Autodesk Inventor part; units mm, degrees
(part 2 of 2)
sketch "Sketch100" plane through (-49.2721, -156.6302, 132.2833) normal (0, -0.6427876, 0.7660444) x (1, 0, 0)
  line L0 (3.9589, -29.4362) -> (45.851, -29.4362) construction
  line L1 (45.851, -29.4362) -> (45.851, -41.0729) construction
  line L2 (45.851, -41.0729) -> (3.9589, -41.0729) construction
  line L3 (3.9589, -41.0729) -> (3.9589, -29.4362) construction
  spline S0 degree 2 poles (6.671, -31.0269) (6.671, -31.4443) (6.3326, -32.1162) (6.0486, -32.3039) knots 0 0 0 1 2 2 2
  spline S1 degree 2 poles (6.0486, -32.3039) (5.8164, -32.4496) (5.3397, -32.5484) (4.9692, -32.5484) knots 0 0 0 1 2 2 2
  line L4 (4.9692, -32.5484) -> (4.2677, -32.5484)
  line L5 (4.2677, -32.5484) -> (4.2677, -29.5004)
  line L6 (4.2677, -29.5004) -> (4.9617, -29.5004)
  spline S2 degree 2 poles (4.9617, -29.5004) (5.3915, -29.5004) (5.8806, -29.6289) (6.0535, -29.7425) knots 0 0 0 1 2 2 2
  spline S3 degree 2 poles (6.0535, -29.7425) (6.3474, -29.9376) (6.671, -30.5823) (6.671, -31.0269) knots 0 0 0 1 2 2 2
  spline S4 degree 2 poles (6.2486, -31.0219) (6.2486, -30.6712) (6.0164, -30.1747) (5.7867, -30.0339) knots 0 0 0 1 2 2 2
  spline S5 degree 2 poles (5.7867, -30.0339) (5.6237, -29.9376) (5.2557, -29.8512) (4.9815, -29.8512) knots 0 0 0 1 2 2 2
  line L7 (4.9815, -29.8512) -> (4.6728, -29.8512)
  line L8 (4.6728, -29.8512) -> (4.6728, -32.1977)
  line L9 (4.6728, -32.1977) -> (4.9815, -32.1977)
  spline S6 degree 2 poles (4.9815, -32.1977) (5.2507, -32.1977) (5.6583, -32.1112) (5.8238, -31.9951) knots 0 0 0 1 2 2 2
  spline S7 degree 2 poles (5.8238, -31.9951) (6.0362, -31.8519) (6.2486, -31.3776) (6.2486, -31.0219) knots 0 0 0 1 2 2 2
  spline S8 degree 2 poles (8.1752, -32.6126) (7.906, -32.6126) (7.5059, -32.4718) (7.3651, -32.331) knots 0 0 0 1 2 2 2
  spline S9 degree 2 poles (7.3651, -32.331) (7.2045, -32.173) (7.0736, -31.7284) (7.0736, -31.4023) knots 0 0 0 1 2 2 2
  line L10 (7.0736, -31.4023) -> (7.0736, -29.5004)
  line L11 (7.0736, -29.5004) -> (7.4787, -29.5004)
  line L12 (7.4787, -29.5004) -> (7.4787, -31.4023)
  spline S10 degree 2 poles (7.4787, -31.4023) (7.4787, -31.6147) (7.533, -31.9013) (7.6096, -32.0174) knots 0 0 0 1 2 2 2
  spline S11 degree 2 poles (7.6096, -32.0174) (7.6911, -32.1409) (7.9727, -32.2668) (8.1752, -32.2668) knots 0 0 0 1 2 2 2
  spline S12 degree 2 poles (8.1752, -32.2668) (8.3654, -32.2668) (8.6618, -32.1409) (8.7433, -32.0174) knots 0 0 0 1 2 2 2
  spline S13 degree 2 poles (8.7433, -32.0174) (8.8199, -31.9013) (8.8743, -31.6172) (8.8743, -31.4122) knots 0 0 0 1 2 2 2
  line L13 (8.8743, -31.4122) -> (8.8743, -29.5004)
  line L14 (8.8743, -29.5004) -> (9.2793, -29.5004)
  line L15 (9.2793, -29.5004) -> (9.2793, -31.4023)
  spline S14 degree 2 poles (9.2793, -31.4023) (9.2793, -31.721) (9.1509, -32.1754) (8.9879, -32.331) knots 0 0 0 1 2 2 2
  spline S15 degree 2 poles (8.9879, -32.331) (8.8421, -32.4743) (8.4568, -32.6126) (8.1752, -32.6126) knots 0 0 0 1 2 2 2
  line L16 (9.5313, -32.5484) -> (10.5588, -29.5004)
  line L17 (10.5588, -29.5004) -> (11.0577, -29.5004)
  line L18 (11.0577, -29.5004) -> (12.0853, -32.5484)
  line L19 (12.0853, -32.5484) -> (11.658, -32.5484)
  line L20 (11.658, -32.5484) -> (11.3813, -31.6963)
  line L21 (11.3813, -31.6963) -> (10.2179, -31.6963)
  line L22 (10.2179, -31.6963) -> (9.9413, -32.5484)
  line L23 (9.9413, -32.5484) -> (9.5313, -32.5484)
  line L24 (11.2702, -31.3505) -> (10.7984, -29.9154)
  line L25 (10.7984, -29.9154) -> (10.3291, -31.3505)
  line L26 (10.3291, -31.3505) -> (11.2702, -31.3505)
  line L27 (14.1403, -32.5484) -> (12.3743, -32.5484)
  line L28 (12.3743, -32.5484) -> (12.3743, -29.5004)
  line L29 (12.3743, -29.5004) -> (12.7793, -29.5004)
  line L30 (12.7793, -29.5004) -> (12.7793, -32.1878)
  line L31 (12.7793, -32.1878) -> (14.1403, -32.1878)
  line L32 (14.1403, -32.1878) -> (14.1403, -32.5484)
  line L33 (17.9787, -29.5004) -> (16.929, -32.5484)
  line L34 (16.929, -32.5484) -> (16.4918, -32.5484)
  line L35 (16.4918, -32.5484) -> (15.442, -29.5004)
  line L36 (15.442, -29.5004) -> (15.8767, -29.5004)
  line L37 (15.8767, -29.5004) -> (16.7215, -32.0322)
  line L38 (16.7215, -32.0322) -> (17.5662, -29.5004)
  line L39 (17.5662, -29.5004) -> (17.9787, -29.5004)
  line L40 (19.3323, -32.5484) -> (18.1516, -32.5484)
  line L41 (18.1516, -32.5484) -> (18.1516, -32.2372)
  line L42 (18.1516, -32.2372) -> (18.5394, -32.2372)
  line L43 (18.5394, -32.2372) -> (18.5394, -29.8116)
  line L44 (18.5394, -29.8116) -> (18.1516, -29.8116)
  line L45 (18.1516, -29.8116) -> (18.1516, -29.5004)
  line L46 (18.1516, -29.5004) -> (19.3323, -29.5004)
  line L47 (19.3323, -29.5004) -> (19.3323, -29.8116)
  line L48 (19.3323, -29.8116) -> (18.9445, -29.8116)
  line L49 (18.9445, -29.8116) -> (18.9445, -32.2372)
  line L50 (18.9445, -32.2372) -> (19.3323, -32.2372)
  line L51 (19.3323, -32.2372) -> (19.3323, -32.5484)
  spline S16 degree 2 poles (20.6834, -32.6028) (20.3524, -32.6028) (19.8881, -32.4644) (19.683, -32.3656) knots 0 0 0 1 2 2 2
  line L52 (19.683, -32.3656) -> (19.683, -31.8568)
  line L53 (19.683, -31.8568) -> (19.7127, -31.8568)
  spline S17 degree 2 poles (19.7127, -31.8568) (19.9128, -32.0445) (20.4191, -32.252) (20.6538, -32.252) knots 0 0 0 1 2 2 2
  spline S18 degree 2 poles (20.6538, -32.252) (20.9897, -32.252) (21.333, -31.9729) (21.333, -31.7432) knots 0 0 0 1 2 2 2
  spline S19 degree 2 poles (21.333, -31.7432) (21.333, -31.5604) (21.1527, -31.3332) (20.9576, -31.2764) knots 0 0 0 1 2 2 2
  spline S20 degree 2 poles (20.9576, -31.2764) (20.8168, -31.2368) (20.5821, -31.1825) (20.4068, -31.138) knots 0 0 0 1 2 2 2
  spline S21 degree 2 poles (20.4068, -31.138) (20.2487, -31.096) (19.9992, -30.9701) (19.9029, -30.8688) knots 0 0 0 1 2 2 2
  spline S22 degree 2 poles (19.9029, -30.8688) (19.809, -30.7675) (19.7053, -30.4958) (19.7053, -30.318) knots 0 0 0 1 2 2 2
  spline S23 degree 2 poles (19.7053, -30.318) (19.7053, -29.9475) (20.2833, -29.4461) (20.7303, -29.4461) knots 0 0 0 1 2 2 2
  spline S24 degree 2 poles (20.7303, -29.4461) (20.9872, -29.4461) (21.4417, -29.5473) (21.6368, -29.6437) knots 0 0 0 1 2 2 2
  line L54 (21.6368, -29.6437) -> (21.6368, -30.1278)
  line L55 (21.6368, -30.1278) -> (21.6072, -30.1278)
  spline S25 degree 2 poles (21.6072, -30.1278) (21.4615, -29.9944) (21.007, -29.7968) (20.7575, -29.7968) knots 0 0 0 1 2 2 2
  spline S26 degree 2 poles (20.7575, -29.7968) (20.4759, -29.7968) (20.1276, -30.0611) (20.1276, -30.276) knots 0 0 0 1 2 2 2
  spline S27 degree 2 poles (20.1276, -30.276) (20.1276, -30.4687) (20.3327, -30.6984) (20.5253, -30.7502) knots 0 0 0 1 2 2 2
  spline S28 degree 2 poles (20.5253, -30.7502) (20.6538, -30.7848) (21.0267, -30.8737) (21.1502, -30.9108) knots 0 0 0 1 2 2 2
  spline S29 degree 2 poles (21.1502, -30.9108) (21.4639, -31.0071) (21.7554, -31.3949) (21.7554, -31.679) knots 0 0 0 1 2 2 2
  spline S30 degree 2 poles (21.7554, -31.679) (21.7554, -31.8593) (21.6097, -32.2051) (21.4787, -32.3261) knots 0 0 0 1 2 2 2
  spline S31 degree 2 poles (21.4787, -32.3261) (21.333, -32.4595) (20.9625, -32.6028) (20.6834, -32.6028) knots 0 0 0 1 2 2 2
  line L56 (23.23, -32.5484) -> (22.0493, -32.5484)
  line L57 (22.0493, -32.5484) -> (22.0493, -32.2372)
  line L58 (22.0493, -32.2372) -> (22.4371, -32.2372)
  line L59 (22.4371, -32.2372) -> (22.4371, -29.8116)
  line L60 (22.4371, -29.8116) -> (22.0493, -29.8116)
  line L61 (22.0493, -29.8116) -> (22.0493, -29.5004)
  line L62 (22.0493, -29.5004) -> (23.23, -29.5004)
  line L63 (23.23, -29.5004) -> (23.23, -29.8116)
  line L64 (23.23, -29.8116) -> (22.8422, -29.8116)
  line L65 (22.8422, -29.8116) -> (22.8422, -32.2372)
  line L66 (22.8422, -32.2372) -> (23.23, -32.2372)
  line L67 (23.23, -32.2372) -> (23.23, -32.5484)
  spline S32 degree 2 poles (25.8877, -29.8487) (26.0606, -30.0512) (26.2533, -30.644) (26.2533, -31.0244) knots 0 0 0 1 2 2 2
  spline S33 degree 2 poles (26.2533, -31.0244) (26.2533, -31.3949) (26.0656, -31.9951) (25.8877, -32.1977) knots 0 0 0 1 2 2 2
  spline S34 degree 2 poles (25.8877, -32.1977) (25.7, -32.4101) (25.2035, -32.6126) (24.9047, -32.6126) knots 0 0 0 1 2 2 2
  spline S35 degree 2 poles (24.9047, -32.6126) (24.5959, -32.6126) (24.1019, -32.4027) (23.9216, -32.1977) knots 0 0 0 1 2 2 2
  spline S36 degree 2 poles (23.9216, -32.1977) (23.7462, -31.9951) (23.5585, -31.3999) (23.5585, -31.0244) knots 0 0 0 1 2 2 2
  spline S37 degree 2 poles (23.5585, -31.0244) (23.5585, -30.6416) (23.7487, -30.0586) (23.9241, -29.8487) knots 0 0 0 1 2 2 2
  spline S38 degree 2 poles (23.9241, -29.8487) (24.1019, -29.6461) (24.5984, -29.4362) (24.9047, -29.4362) knots 0 0 0 1 2 2 2
  spline S39 degree 2 poles (24.9047, -29.4362) (25.2159, -29.4362) (25.7148, -29.6536) (25.8877, -29.8487) knots 0 0 0 1 2 2 2
  spline S40 degree 2 poles (25.8309, -31.0244) (25.8309, -30.7231) (25.7, -30.2562) (25.5814, -30.1031) knots 0 0 0 1 2 2 2
  spline S41 degree 2 poles (25.5814, -30.1031) (25.4604, -29.945) (25.1195, -29.7869) (24.9071, -29.7869) knots 0 0 0 1 2 2 2
  spline S42 degree 2 poles (24.9071, -29.7869) (24.6873, -29.7869) (24.3563, -29.9401) (24.2303, -30.1031) knots 0 0 0 1 2 2 2
  spline S43 degree 2 poles (24.2303, -30.1031) (24.1093, -30.2587) (23.9809, -30.728) (23.9809, -31.0244) knots 0 0 0 1 2 2 2
  spline S44 degree 2 poles (23.9809, -31.0244) (23.9809, -31.6246) (24.4848, -32.2619) (24.9071, -32.2619) knots 0 0 0 1 2 2 2
  spline S45 degree 2 poles (24.9071, -32.2619) (25.3295, -32.2619) (25.8309, -31.6246) (25.8309, -31.0244) knots 0 0 0 1 2 2 2
  line L68 (28.8789, -32.5484) -> (28.4244, -32.5484)
  line L69 (28.4244, -32.5484) -> (27.0758, -29.9203)
  line L70 (27.0758, -29.9203) -> (27.0758, -32.5484)
  line L71 (27.0758, -32.5484) -> (26.6979, -32.5484)
  line L72 (26.6979, -32.5484) -> (26.6979, -29.5004)
  line L73 (26.6979, -29.5004) -> (27.2734, -29.5004)
  line L74 (27.2734, -29.5004) -> (28.501, -31.9136)
  line L75 (28.501, -31.9136) -> (28.501, -29.5004)
  line L76 (28.501, -29.5004) -> (28.8789, -29.5004)
  line L77 (28.8789, -29.5004) -> (28.8789, -32.5484)
  line L78 (33.0187, -32.5484) -> (32.6136, -32.5484)
  line L79 (32.6136, -32.5484) -> (32.6136, -31.0565)
  line L80 (32.6136, -31.0565) -> (31.2106, -31.0565)
  line L81 (31.2106, -31.0565) -> (31.2106, -32.5484)
  line L82 (31.2106, -32.5484) -> (30.8055, -32.5484)
  line L83 (30.8055, -32.5484) -> (30.8055, -29.5004)
  line L84 (30.8055, -29.5004) -> (31.2106, -29.5004)
  line L85 (31.2106, -29.5004) -> (31.2106, -30.6959)
  line L86 (31.2106, -30.6959) -> (32.6136, -30.6959)
  line L87 (32.6136, -30.6959) -> (32.6136, -29.5004)
  line L88 (32.6136, -29.5004) -> (33.0187, -29.5004)
  line L89 (33.0187, -29.5004) -> (33.0187, -32.5484)
  spline S46 degree 2 poles (35.7925, -29.8487) (35.9654, -30.0512) (36.1581, -30.644) (36.1581, -31.0244) knots 0 0 0 1 2 2 2
  spline S47 degree 2 poles (36.1581, -31.0244) (36.1581, -31.3949) (35.9703, -31.9951) (35.7925, -32.1977) knots 0 0 0 1 2 2 2
  spline S48 degree 2 poles (35.7925, -32.1977) (35.6048, -32.4101) (35.1083, -32.6126) (34.8094, -32.6126) knots 0 0 0 1 2 2 2
  spline S49 degree 2 poles (34.8094, -32.6126) (34.5007, -32.6126) (34.0067, -32.4027) (33.8264, -32.1977) knots 0 0 0 1 2 2 2
  spline S50 degree 2 poles (33.8264, -32.1977) (33.651, -31.9951) (33.4633, -31.3999) (33.4633, -31.0244) knots 0 0 0 1 2 2 2
  spline S51 degree 2 poles (33.4633, -31.0244) (33.4633, -30.6416) (33.6535, -30.0586) (33.8288, -29.8487) knots 0 0 0 1 2 2 2
  spline S52 degree 2 poles (33.8288, -29.8487) (34.0067, -29.6461) (34.5031, -29.4362) (34.8094, -29.4362) knots 0 0 0 1 2 2 2
  spline S53 degree 2 poles (34.8094, -29.4362) (35.1206, -29.4362) (35.6196, -29.6536) (35.7925, -29.8487) knots 0 0 0 1 2 2 2
  spline S54 degree 2 poles (35.7357, -31.0244) (35.7357, -30.7231) (35.6048, -30.2562) (35.4862, -30.1031) knots 0 0 0 1 2 2 2
  spline S55 degree 2 poles (35.4862, -30.1031) (35.3652, -29.945) (35.0243, -29.7869) (34.8119, -29.7869) knots 0 0 0 1 2 2 2
  spline S56 degree 2 poles (34.8119, -29.7869) (34.5921, -29.7869) (34.2611, -29.9401) (34.1351, -30.1031) knots 0 0 0 1 2 2 2
  spline S57 degree 2 poles (34.1351, -30.1031) (34.0141, -30.2587) (33.8856, -30.728) (33.8856, -31.0244) knots 0 0 0 1 2 2 2
  spline S58 degree 2 poles (33.8856, -31.0244) (33.8856, -31.6246) (34.3895, -32.2619) (34.8119, -32.2619) knots 0 0 0 1 2 2 2
  spline S59 degree 2 poles (34.8119, -32.2619) (35.2343, -32.2619) (35.7357, -31.6246) (35.7357, -31.0244) knots 0 0 0 1 2 2 2
  line L90 (38.3687, -32.5484) -> (36.6027, -32.5484)
  line L91 (36.6027, -32.5484) -> (36.6027, -29.5004)
  line L92 (36.6027, -29.5004) -> (37.0077, -29.5004)
  line L93 (37.0077, -29.5004) -> (37.0077, -32.1878)
  line L94 (37.0077, -32.1878) -> (38.3687, -32.1878)
  line L95 (38.3687, -32.1878) -> (38.3687, -32.5484)
  spline S60 degree 2 poles (41.0907, -31.0269) (41.0907, -31.4443) (40.7523, -32.1162) (40.4682, -32.3039) knots 0 0 0 1 2 2 2
  spline S61 degree 2 poles (40.4682, -32.3039) (40.236, -32.4496) (39.7593, -32.5484) (39.3888, -32.5484) knots 0 0 0 1 2 2 2
  line L96 (39.3888, -32.5484) -> (38.6873, -32.5484)
  line L97 (38.6873, -32.5484) -> (38.6873, -29.5004)
  line L98 (38.6873, -29.5004) -> (39.3814, -29.5004)
  spline S62 degree 2 poles (39.3814, -29.5004) (39.8112, -29.5004) (40.3003, -29.6289) (40.4732, -29.7425) knots 0 0 0 1 2 2 2
  spline S63 degree 2 poles (40.4732, -29.7425) (40.7671, -29.9376) (41.0907, -30.5823) (41.0907, -31.0269) knots 0 0 0 1 2 2 2
  spline S64 degree 2 poles (40.6683, -31.0219) (40.6683, -30.6712) (40.4361, -30.1747) (40.2064, -30.0339) knots 0 0 0 1 2 2 2
  spline S65 degree 2 poles (40.2064, -30.0339) (40.0434, -29.9376) (39.6754, -29.8512) (39.4012, -29.8512) knots 0 0 0 1 2 2 2
  line L99 (39.4012, -29.8512) -> (39.0924, -29.8512)
  line L100 (39.0924, -29.8512) -> (39.0924, -32.1977)
  line L101 (39.0924, -32.1977) -> (39.4012, -32.1977)
  spline S66 degree 2 poles (39.4012, -32.1977) (39.6704, -32.1977) (40.078, -32.1112) (40.2435, -31.9951) knots 0 0 0 1 2 2 2
  spline S67 degree 2 poles (40.2435, -31.9951) (40.4559, -31.8519) (40.6683, -31.3776) (40.6683, -31.0219) knots 0 0 0 1 2 2 2
  line L102 (41.5303, -32.5484) -> (41.5303, -29.5004)
  line L103 (41.5303, -29.5004) -> (43.4372, -29.5004)
  line L104 (43.4372, -29.5004) -> (43.4372, -29.861)
  line L105 (43.4372, -29.861) -> (41.9354, -29.861)
  line L106 (41.9354, -29.861) -> (41.9354, -30.6959)
  line L107 (41.9354, -30.6959) -> (43.3359, -30.6959)
  line L108 (43.3359, -30.6959) -> (43.3359, -31.0565)
  line L109 (43.3359, -31.0565) -> (41.9354, -31.0565)
  line L110 (41.9354, -31.0565) -> (41.9354, -32.1878)
  line L111 (41.9354, -32.1878) -> (43.4372, -32.1878)
  line L112 (43.4372, -32.1878) -> (43.4372, -32.5484)
  line L113 (43.4372, -32.5484) -> (41.5303, -32.5484)
  line L114 (46.2407, -32.5484) -> (45.7145, -32.5484)
  line L115 (45.7145, -32.5484) -> (44.7512, -31.3356)
  line L116 (44.7512, -31.3356) -> (44.2869, -31.3356)
  line L117 (44.2869, -31.3356) -> (44.2869, -32.5484)
  line L118 (44.2869, -32.5484) -> (43.8818, -32.5484)
  line L119 (43.8818, -32.5484) -> (43.8818, -29.5004)
  line L120 (43.8818, -29.5004) -> (44.6673, -29.5004)
  spline S68 degree 2 poles (44.6673, -29.5004) (44.9291, -29.5004) (45.2823, -29.5572) (45.4428, -29.661) knots 0 0 0 1 2 2 2
  spline S69 degree 2 poles (45.4428, -29.661) (45.6034, -29.7647) (45.7886, -30.0883) (45.7886, -30.3279) knots 0 0 0 1 2 2 2
  spline S70 degree 2 poles (45.7886, -30.3279) (45.7886, -30.6613) (45.4478, -31.1133) (45.1563, -31.222) knots 0 0 0 1 2 2 2
  line L121 (45.1563, -31.222) -> (46.2407, -32.5484)
  spline S71 degree 2 poles (45.3663, -30.36) (45.3663, -30.2266) (45.2724, -30.0216) (45.1736, -29.9549) knots 0 0 0 1 2 2 2
  spline S72 degree 2 poles (45.1736, -29.9549) (45.0872, -29.8981) (44.8574, -29.8512) (44.6895, -29.8512) knots 0 0 0 1 2 2 2
  line L122 (44.6895, -29.8512) -> (44.2869, -29.8512)
  line L123 (44.2869, -29.8512) -> (44.2869, -30.9972)
  line L124 (44.2869, -30.9972) -> (44.6426, -30.9972)
  spline S73 degree 2 poles (44.6426, -30.9972) (44.8179, -30.9972) (45.097, -30.9355) (45.1934, -30.8392) knots 0 0 0 1 2 2 2
  spline S74 degree 2 poles (45.1934, -30.8392) (45.2823, -30.7552) (45.3663, -30.5181) (45.3663, -30.36) knots 0 0 0 1 2 2 2
  spline S75 degree 2 poles (6.0782, -36.0429) (6.0782, -36.8629) (5.6015, -37.6311) (5.105, -37.6311) knots 0 0 0 1 2 2 2
  spline S76 degree 2 poles (5.105, -37.6311) (4.6011, -37.6311) (4.1294, -36.8481) (4.1294, -36.0453) knots 0 0 0 1 2 2 2
  spline S77 degree 2 poles (4.1294, -36.0453) (4.1294, -35.2203) (4.6061, -34.4571) (5.105, -34.4571) knots 0 0 0 1 2 2 2
  spline S78 degree 2 poles (5.105, -34.4571) (5.6064, -34.4571) (6.0782, -35.2475) (6.0782, -36.0429) knots 0 0 0 1 2 2 2
  spline S79 degree 2 poles (5.5546, -36.9716) (5.6138, -36.8209) (5.6632, -36.3566) (5.6632, -36.0429) knots 0 0 0 1 2 2 2
  spline S80 degree 2 poles (5.6632, -36.0429) (5.6632, -35.7292) (5.6138, -35.2673) (5.5521, -35.1117) knots 0 0 0 1 2 2 2
  spline S81 degree 2 poles (5.5521, -35.1117) (5.4903, -34.9561) (5.2754, -34.7955) (5.105, -34.7955) knots 0 0 0 1 2 2 2
  spline S82 degree 2 poles (5.105, -34.7955) (4.9346, -34.7955) (4.7147, -34.9561) (4.6505, -35.1166) knots 0 0 0 1 2 2 2
  spline S83 degree 2 poles (4.6505, -35.1166) (4.5888, -35.2722) (4.5443, -35.7465) (4.5443, -36.0453) knots 0 0 0 1 2 2 2
  spline S84 degree 2 poles (4.5443, -36.0453) (4.5443, -36.3664) (4.5838, -36.7962) (4.6481, -36.9642) knots 0 0 0 1 2 2 2
  spline S85 degree 2 poles (4.6481, -36.9642) (4.7073, -37.1223) (4.9272, -37.2927) (5.105, -37.2927) knots 0 0 0 1 2 2 2
  spline S86 degree 2 poles (5.105, -37.2927) (5.273, -37.2927) (5.4928, -37.1321) (5.5546, -36.9716) knots 0 0 0 1 2 2 2
  spline S87 degree 2 poles (7.3898, -37.636) (7.1625, -37.636) (6.7896, -37.5002) (6.6586, -37.3742) knots 0 0 0 1 2 2 2
  spline S88 degree 2 poles (6.6586, -37.3742) (6.5302, -37.2507) (6.3968, -36.9148) (6.3968, -36.7246) knots 0 0 0 1 2 2 2
  spline S89 degree 2 poles (6.3968, -36.7246) (6.3968, -36.4776) (6.6611, -36.0626) (6.9131, -35.9391) knots 0 0 0 1 2 2 2
  line L125 (6.9131, -35.9391) -> (6.9131, -35.9268)
  spline S90 degree 2 poles (6.9131, -35.9268) (6.6883, -35.7959) (6.4709, -35.4846) (6.4709, -35.2525) knots 0 0 0 1 2 2 2
  spline S91 degree 2 poles (6.4709, -35.2525) (6.4709, -34.9091) (6.9896, -34.4497) (7.3898, -34.4497) knots 0 0 0 1 2 2 2
  spline S92 degree 2 poles (7.3898, -34.4497) (7.8047, -34.4497) (8.3061, -34.8844) (8.3061, -35.2253) knots 0 0 0 1 2 2 2
  spline S93 degree 2 poles (8.3061, -35.2253) (8.3061, -35.4303) (8.0666, -35.8304) (7.8418, -35.9441) knots 0 0 0 1 2 2 2
  line L126 (7.8418, -35.9441) -> (7.8418, -35.9564)
  spline S94 degree 2 poles (7.8418, -35.9564) (8.1085, -36.0799) (8.3827, -36.4356) (8.3827, -36.7172) knots 0 0 0 1 2 2 2
  spline S95 degree 2 poles (8.3827, -36.7172) (8.3827, -37.1074) (7.8146, -37.636) (7.3898, -37.636) knots 0 0 0 1 2 2 2
  spline S96 degree 2 poles (7.9628, -36.7567) (7.9628, -36.569) (7.8146, -36.3467) (7.6047, -36.2331) knots 0 0 0 1 2 2 2
  spline S97 degree 2 poles (7.6047, -36.2331) (7.5355, -36.1935) (7.3033, -36.1021) (7.1576, -36.0429) knots 0 0 0 1 2 2 2
  spline S98 degree 2 poles (7.1576, -36.0429) (6.9896, -36.154) (6.8093, -36.485) (6.8093, -36.6949) knots 0 0 0 1 2 2 2
  spline S99 degree 2 poles (6.8093, -36.6949) (6.8093, -36.9716) (7.1428, -37.3322) (7.3947, -37.3322) knots 0 0 0 1 2 2 2
  spline S100 degree 2 poles (7.3947, -37.3322) (7.6516, -37.3322) (7.9628, -37.0235) (7.9628, -36.7567) knots 0 0 0 1 2 2 2
  spline S101 degree 2 poles (7.906, -35.2302) (7.906, -35.0252) (7.6318, -34.751) (7.3873, -34.751) knots 0 0 0 1 2 2 2
  spline S102 degree 2 poles (7.3873, -34.751) (7.165, -34.751) (6.8809, -34.9956) (6.8809, -35.2055) knots 0 0 0 1 2 2 2
  spline S103 degree 2 poles (6.8809, -35.2055) (6.8809, -35.3562) (7.0267, -35.5661) (7.1724, -35.6501) knots 0 0 0 1 2 2 2
  spline S104 degree 2 poles (7.1724, -35.6501) (7.2342, -35.6847) (7.496, -35.8057) (7.6022, -35.8403) knots 0 0 0 1 2 2 2
  spline S105 degree 2 poles (7.6022, -35.8403) (7.78, -35.7045) (7.906, -35.4155) (7.906, -35.2302) knots 0 0 0 1 2 2 2
  line L127 (9.4102, -37.5669) -> (8.9212, -37.5669)
  line L128 (8.9212, -37.5669) -> (8.9212, -36.9839)
  line L129 (8.9212, -36.9839) -> (9.4102, -36.9839)
  line L130 (9.4102, -36.9839) -> (9.4102, -37.5669)
  line L131 (11.905, -37.5669) -> (10.0253, -37.5669)
  line L132 (10.0253, -37.5669) -> (10.0253, -37.1346)
  spline S106 degree 2 poles (10.0253, -37.1346) (10.2278, -36.9444) (10.5884, -36.5912) (10.7613, -36.401) knots 0 0 0 1 2 2 2
  spline S107 degree 2 poles (10.7613, -36.401) (11.1096, -36.0182) (11.364, -35.5587) (11.364, -35.3142) knots 0 0 0 1 2 2 2
  spline S108 degree 2 poles (11.364, -35.3142) (11.364, -35.1858) (11.285, -34.9931) (11.2134, -34.9314) knots 0 0 0 1 2 2 2
  spline S109 degree 2 poles (11.2134, -34.9314) (11.1417, -34.8696) (10.954, -34.8079) (10.8404, -34.8079) knots 0 0 0 1 2 2 2
  spline S110 degree 2 poles (10.8404, -34.8079) (10.7317, -34.8079) (10.5094, -34.8622) (10.4081, -34.9042) knots 0 0 0 1 2 2 2
  spline S111 degree 2 poles (10.4081, -34.9042) (10.3217, -34.9388) (10.1611, -35.0376) (10.1117, -35.0721) knots 0 0 0 1 2 2 2
  line L133 (10.1117, -35.0721) -> (10.0895, -35.0721)
  line L134 (10.0895, -35.0721) -> (10.0895, -34.6374)
  spline S112 degree 2 poles (10.0895, -34.6374) (10.2155, -34.5757) (10.6675, -34.4546) (10.87, -34.4546) knots 0 0 0 1 2 2 2
  spline S113 degree 2 poles (10.87, -34.4546) (11.2973, -34.4546) (11.779, -34.9067) (11.779, -35.292) knots 0 0 0 1 2 2 2
  spline S114 degree 2 poles (11.779, -35.292) (11.779, -35.4723) (11.695, -35.7736) (11.6209, -35.9021) knots 0 0 0 1 2 2 2
  spline S115 degree 2 poles (11.6209, -35.9021) (11.5468, -36.0355) (11.3319, -36.2973) (11.2134, -36.4232) knots 0 0 0 1 2 2 2
  spline S116 degree 2 poles (11.2134, -36.4232) (11.0207, -36.6332) (10.5489, -37.0827) (10.4081, -37.2137) knots 0 0 0 1 2 2 2
  line L135 (10.4081, -37.2137) -> (11.905, -37.2137)
  line L136 (11.905, -37.2137) -> (11.905, -37.5669)
  spline S117 degree 2 poles (14.1601, -36.5986) (14.1601, -36.8184) (14.0193, -37.1939) (13.8909, -37.3322) knots 0 0 0 1 2 2 2
  spline S118 degree 2 poles (13.8909, -37.3322) (13.7624, -37.4705) (13.3796, -37.6311) (13.1424, -37.6311) knots 0 0 0 1 2 2 2
  spline S119 degree 2 poles (13.1424, -37.6311) (12.9251, -37.6311) (12.5002, -37.5348) (12.3446, -37.4582) knots 0 0 0 1 2 2 2
  line L137 (12.3446, -37.4582) -> (12.3446, -37.0259)
  line L138 (12.3446, -37.0259) -> (12.3743, -37.0259)
  spline S120 degree 2 poles (12.3743, -37.0259) (12.4212, -37.0605) (12.5966, -37.1494) (12.7028, -37.189) knots 0 0 0 1 2 2 2
  spline S121 degree 2 poles (12.7028, -37.189) (12.8238, -37.2309) (13.0239, -37.2779) (13.1499, -37.2779) knots 0 0 0 1 2 2 2
  spline S122 degree 2 poles (13.1499, -37.2779) (13.2734, -37.2779) (13.5055, -37.189) (13.5895, -37.0926) knots 0 0 0 1 2 2 2
  spline S123 degree 2 poles (13.5895, -37.0926) (13.6661, -37.0012) (13.7451, -36.7592) (13.7451, -36.5961) knots 0 0 0 1 2 2 2
  spline S124 degree 2 poles (13.7451, -36.5961) (13.7451, -36.4331) (13.6562, -36.2256) (13.5722, -36.1565) knots 0 0 0 1 2 2 2
  spline S125 degree 2 poles (13.5722, -36.1565) (13.4858, -36.0799) (13.2289, -36.0157) (13.0733, -36.0157) knots 0 0 0 1 2 2 2
  spline S126 degree 2 poles (13.0733, -36.0157) (12.9053, -36.0157) (12.5719, -36.0676) (12.4706, -36.0898) knots 0 0 0 1 2 2 2
  line L139 (12.4706, -36.0898) -> (12.4706, -34.5189)
  line L140 (12.4706, -34.5189) -> (14.1428, -34.5189)
  line L141 (14.1428, -34.5189) -> (14.1428, -34.877)
  line L142 (14.1428, -34.877) -> (12.8633, -34.877)
  line L143 (12.8633, -34.877) -> (12.8633, -35.6897)
  spline S127 degree 2 poles (12.8633, -35.6897) (12.9374, -35.6798) (13.0807, -35.6724) (13.14, -35.6724) knots 0 0 0 1 2 2 2
  spline S128 degree 2 poles (13.14, -35.6724) (13.3746, -35.6724) (13.6982, -35.7489) (13.8464, -35.8626) knots 0 0 0 1 2 2 2
  spline S129 degree 2 poles (13.8464, -35.8626) (13.9971, -35.9762) (14.1601, -36.322) (14.1601, -36.5986) knots 0 0 0 1 2 2 2
  line L144 (15.2543, -37.5669) -> (14.7652, -37.5669)
  line L145 (14.7652, -37.5669) -> (14.7652, -36.9839)
  line L146 (14.7652, -36.9839) -> (15.2543, -36.9839)
  line L147 (15.2543, -36.9839) -> (15.2543, -37.5669)
  line L148 (17.749, -37.5669) -> (15.8693, -37.5669)
  line L149 (15.8693, -37.5669) -> (15.8693, -37.1346)
  spline S130 degree 2 poles (15.8693, -37.1346) (16.0719, -36.9444) (16.4325, -36.5912) (16.6054, -36.401) knots 0 0 0 1 2 2 2
  spline S131 degree 2 poles (16.6054, -36.401) (16.9537, -36.0182) (17.2081, -35.5587) (17.2081, -35.3142) knots 0 0 0 1 2 2 2
  spline S132 degree 2 poles (17.2081, -35.3142) (17.2081, -35.1858) (17.129, -34.9931) (17.0574, -34.9314) knots 0 0 0 1 2 2 2
  spline S133 degree 2 poles (17.0574, -34.9314) (16.9858, -34.8696) (16.7981, -34.8079) (16.6844, -34.8079) knots 0 0 0 1 2 2 2
  spline S134 degree 2 poles (16.6844, -34.8079) (16.5758, -34.8079) (16.3535, -34.8622) (16.2522, -34.9042) knots 0 0 0 1 2 2 2
  spline S135 degree 2 poles (16.2522, -34.9042) (16.1657, -34.9388) (16.0052, -35.0376) (15.9558, -35.0721) knots 0 0 0 1 2 2 2
  line L150 (15.9558, -35.0721) -> (15.9336, -35.0721)
  line L151 (15.9336, -35.0721) -> (15.9336, -34.6374)
  spline S136 degree 2 poles (15.9336, -34.6374) (16.0595, -34.5757) (16.5115, -34.4546) (16.7141, -34.4546) knots 0 0 0 1 2 2 2
  spline S137 degree 2 poles (16.7141, -34.4546) (17.1414, -34.4546) (17.6231, -34.9067) (17.6231, -35.292) knots 0 0 0 1 2 2 2
  spline S138 degree 2 poles (17.6231, -35.292) (17.6231, -35.4723) (17.5391, -35.7736) (17.465, -35.9021) knots 0 0 0 1 2 2 2
  spline S139 degree 2 poles (17.465, -35.9021) (17.3909, -36.0355) (17.176, -36.2973) (17.0574, -36.4232) knots 0 0 0 1 2 2 2
  spline S140 degree 2 poles (17.0574, -36.4232) (16.8648, -36.6332) (16.393, -37.0827) (16.2522, -37.2137) knots 0 0 0 1 2 2 2
  line L152 (16.2522, -37.2137) -> (17.749, -37.2137)
  line L153 (17.749, -37.2137) -> (17.749, -37.5669)
  spline S141 degree 2 poles (20.0041, -36.5986) (20.0041, -36.8184) (19.8634, -37.1939) (19.7349, -37.3322) knots 0 0 0 1 2 2 2
  spline S142 degree 2 poles (19.7349, -37.3322) (19.6065, -37.4705) (19.2236, -37.6311) (18.9865, -37.6311) knots 0 0 0 1 2 2 2
  spline S143 degree 2 poles (18.9865, -37.6311) (18.7691, -37.6311) (18.3443, -37.5348) (18.1887, -37.4582) knots 0 0 0 1 2 2 2
  line L154 (18.1887, -37.4582) -> (18.1887, -37.0259)
  line L155 (18.1887, -37.0259) -> (18.2183, -37.0259)
  spline S144 degree 2 poles (18.2183, -37.0259) (18.2653, -37.0605) (18.4406, -37.1494) (18.5468, -37.189) knots 0 0 0 1 2 2 2
  spline S145 degree 2 poles (18.5468, -37.189) (18.6679, -37.2309) (18.8679, -37.2779) (18.9939, -37.2779) knots 0 0 0 1 2 2 2
  spline S146 degree 2 poles (18.9939, -37.2779) (19.1174, -37.2779) (19.3496, -37.189) (19.4336, -37.0926) knots 0 0 0 1 2 2 2
  spline S147 degree 2 poles (19.4336, -37.0926) (19.5101, -37.0012) (19.5892, -36.7592) (19.5892, -36.5961) knots 0 0 0 1 2 2 2
  spline S148 degree 2 poles (19.5892, -36.5961) (19.5892, -36.4331) (19.5003, -36.2256) (19.4163, -36.1565) knots 0 0 0 1 2 2 2
  spline S149 degree 2 poles (19.4163, -36.1565) (19.3298, -36.0799) (19.0729, -36.0157) (18.9173, -36.0157) knots 0 0 0 1 2 2 2
  spline S150 degree 2 poles (18.9173, -36.0157) (18.7494, -36.0157) (18.4159, -36.0676) (18.3147, -36.0898) knots 0 0 0 1 2 2 2
  line L156 (18.3147, -36.0898) -> (18.3147, -34.5189)
  line L157 (18.3147, -34.5189) -> (19.9869, -34.5189)
  line L158 (19.9869, -34.5189) -> (19.9869, -34.877)
  line L159 (19.9869, -34.877) -> (18.7074, -34.877)
  line L160 (18.7074, -34.877) -> (18.7074, -35.6897)
  spline S151 degree 2 poles (18.7074, -35.6897) (18.7815, -35.6798) (18.9247, -35.6724) (18.984, -35.6724) knots 0 0 0 1 2 2 2
  spline S152 degree 2 poles (18.984, -35.6724) (19.2187, -35.6724) (19.5423, -35.7489) (19.6905, -35.8626) knots 0 0 0 1 2 2 2
  spline S153 degree 2 poles (19.6905, -35.8626) (19.8411, -35.9762) (20.0041, -36.322) (20.0041, -36.5986) knots 0 0 0 1 2 2 2
  point P0 (49.2721, 34.9556)
  constraints: 2 other
extrude "Extrusion85" cut sketch "Sketch100" against normal blind 2
body "Solid1"
